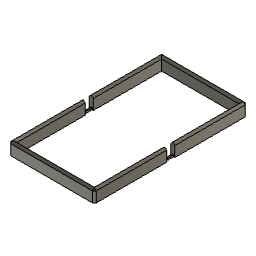
Sifting_Litter_Box_Spacer v3_30mm (Autodesk Fusion 360 design; units mm, degrees)
Autodesk Fusion 360 part; units mm, degrees
sketch "Sketch1" plane through (0, 0, 0) normal (0, 0, 1) x (1, 0, 0)
  line L0 (0, 0) -> (210, 0)
  line L1 (210, 0) -> (210, 355)
  line L2 (210, 355) -> (0, 355)
  line L3 (0, 355) -> (0, 0)
  line L4 (10, 345) -> (10, 10)
  line L5 (10, 10) -> (200, 10)
  line L6 (200, 10) -> (200, 345)
  line L7 (200, 345) -> (10, 345)
  dimension "d4" = 210
  dimension "d5" = 355
  constraint horizontal L0
  constraint vertical L1
  constraint horizontal L2
  constraint vertical L3
  constraint coincident L0.start L3.end
  measures "d4" distance of L0.start L0.end
  measures "d5" distance of L0.start L2.end
extrude "Extrude1" add sketch "Sketch1" along normal blind 30 makes body 1
chamfer "Chamfer1" distance 4.5 angle 45 4 edges at (10, 177.5, 30) (105, 10, 30) (200, 177.5, 30) (105, 345, 30) measured on face at (3.3333, 233.3333, 30) measured on face at (3.3333, 233.3333, 30) measured on face at (3.3333, 233.3333, 30) measured on face at (3.3333, 233.3333, 30) on bodies 1
ref_plane "WorkPlane1" through (105, 177.5, 15) normal (0, -1, 0) x (1, 0, 0)
split "Split1" by plane through (105, 177.5, 15) normal (0, -1, 0) bodies 1 makes body 2 at (70, 0, 10)
move_body "Move1" bodies 1 to x (1, 0, 0) y (0, 1, 0) z (0, 0, 1) at (0, 10, 0)
move_body "Move2" bodies 2 to x (1, 0, 0) y (0, 1, 0) z (0, 0, 1) at (0, -10, 0)
chamfer "Chamfer2" distance 4.5 angle 45 6 edges at (105, 365, 30) (0, 276.25, 30) (210, 276.25, 30) (0, 78.75, 30) (210, 78.75, 30) (105, -10, 30) 6 faces at (140, 365, 10) (0, 305.8333, 20) (210, 246.6667, 20) (0, 108.3333, 20) (210, 49.1667, 20) (70, -10, 10) measured on face at (71.8333, 363.1667, 30) measured on face at (71.8333, 363.1667, 30) measured on face at (71.8333, 363.1667, 30) measured on face at (71.8333, -8.1667, 30) measured on face at (71.8333, -8.1667, 30) measured on face at (71.8333, -8.1667, 30) on bodies 1 2
delete_face "DeleteFace1" 1 faces at (207, 166, 11.5) on bodies 2
delete_face "DeleteFace2" 1 faces at (207, 189, 18.5) on bodies 1
delete_face "DeleteFace3" 1 faces at (3, 189, 18.5) on bodies 1
delete_face "DeleteFace4" 1 faces at (3, 166, 11.5) on bodies 2
delete_face "DeleteFace5" 2 faces at (1.5, 245.1667, 3) (1.5, 52.1667, 3) on bodies 1 2
delete_face "DeleteFace6" 4 faces at (207, 362, 3) (208.5, 302.8333, 3) (207, 109.8333, 1.5) (207, -7, 3) on bodies 1 2
delete_face "DeleteFace7" 1 faces at (140, 362, 1.5) on bodies 1
delete_face "DeleteFace8" 1 faces at (140, -7, 1.5) on bodies 2
delete_face "DeleteFace9" 1 faces at (4.5, 362, 1.5) on bodies 1
delete_face "DeleteFace10" 1 faces at (3, -5.5, 1.5) on bodies 2
delete_face "DeleteFace11" 1 faces at (71.8333, 360.1667, 30) on bodies 1
delete_face "DeleteFace12" 1 faces at (138.1667, -5.1667, 30) on bodies 2
sketch "Sketch2" plane through (0, 187.5, 0) normal (0, -1, 0) x (1, 0, 0)
  line L0 (0, 0) -> (10, 0)
  line L1 (10, 0) -> (10, 25.5)
  line L2 (10, 25.5) -> (5, 30.5)
  line L3 (5, 30.5) -> (0, 25.5)
  line L4 (0, 25.5) -> (0, 0)
  line L5 (3, 0) -> (7, 0)
  line L6 (7, 0) -> (7, 4)
  line L7 (7, 4) -> (3, 4)
  line L8 (3, 4) -> (3, 0)
  dimension "d26" = 4
  dimension "d27" = 4
  constraint horizontal L5
  constraint vertical L6
  constraint horizontal L7
  constraint vertical L8
  constraint coincident L0 L5.start
  measures "d26" distance of L5.start L5.end
  measures "d27" distance of L5.start L7.end
extrude "Extrude2" cut sketch "Sketch2" against normal blind 20 contours L0 L5 L6 L7 L8 bodies 1
sketch "Sketch3" plane through (0, 167.5, 0) normal (0, 1, 0) x (-1, 0, 0)
  line L0 (0, 0) -> (0, 25.5)
  line L1 (0, 25.5) -> (-5, 30.5)
  line L2 (-5, 30.5) -> (-10, 25.5)
  line L3 (-10, 25.5) -> (-10, 0)
  line L4 (-10, 0) -> (0, 0)
  line L5 (-7, 0) -> (-3.2, 0)
  line L6 (-3.2, 0) -> (-3.2, 3.8)
  line L7 (-3.2, 3.8) -> (-7, 3.8)
  line L8 (-7, 3.8) -> (-7, 0)
  dimension "d30" = 3.8
  dimension "d31" = 3.8
  constraint horizontal L5
  constraint vertical L6
  constraint horizontal L7
  constraint vertical L8
  constraint coincident L4 L5.start
  measures "d30" distance of L5.start L5.end
  measures "d31" distance of L5.start L7.end
extrude "Extrude3" add sketch "Sketch3" along normal blind 20 contours L4 L5 L6 L7 L8 bodies 2
sketch "Sketch4" plane through (0, 187.5, 0) normal (0, -1, 0) x (1, 0, 0)
  line L0 (210, 0) -> (210, 25.5)
  line L1 (210, 25.5) -> (205, 30.5)
  line L2 (205, 30.5) -> (200, 25.5)
  line L3 (200, 25.5) -> (200, 0)
  line L4 (200, 0) -> (210, 0)
  line L5 (203, 0) -> (206.8, 0)
  line L6 (206.8, 0) -> (206.8, 3.8)
  line L7 (206.8, 3.8) -> (203, 3.8)
  line L8 (203, 3.8) -> (203, 0)
  dimension "d34" = 3.8
  dimension "d35" = 3.8
  constraint horizontal L5
  constraint vertical L6
  constraint horizontal L7
  constraint vertical L8
  constraint coincident L4 L5.start
  measures "d34" distance of L5.start L5.end
  measures "d35" distance of L5.start L7.end
extrude "Extrude4" add sketch "Sketch4" along normal blind 20 contours L4 L5 L6 L7 L8 bodies 1
sketch "Sketch5" plane through (0, 167.5, 0) normal (0, 1, 0) x (-1, 0, 0)
  line L0 (-210, 0) -> (-200, 0)
  line L1 (-200, 0) -> (-200, 25.5)
  line L2 (-200, 25.5) -> (-205, 30.5)
  line L3 (-205, 30.5) -> (-210, 25.5)
  line L4 (-210, 25.5) -> (-210, 0)
  line L5 (-207, 0) -> (-203, 0)
  line L6 (-203, 0) -> (-203, 4)
  line L7 (-203, 4) -> (-207, 4)
  line L8 (-207, 4) -> (-207, 0)
  dimension "d38" = 4
  dimension "d39" = 4
  constraint horizontal L5
  constraint vertical L6
  constraint horizontal L7
  constraint vertical L8
  constraint coincident L0 L5.start
  measures "d38" distance of L5.start L5.end
  measures "d39" distance of L5.start L7.end
extrude "Extrude5" cut sketch "Sketch5" against normal blind 20 contours L0 L5 L6 L7 L8 bodies 2
equation "Inner_Width = 210 mm"
equation "Inner_Length = 355 mm"
equation "Height = 30 mm"
equation "d4 = Inner_Width"
equation "d5 = Inner_Length"
equation "Thickness = 10 mm"
equation "d7 = -Thickness"
equation "d8 = Height"
equation "Inner_Chamfer = 4.5 mm"
equation "Inner_Chamfer_Angle = 45 deg"
equation "d12 = Inner_Chamfer"
equation "d13 = Inner_Chamfer_Angle"
equation "Outer_Chamfer = 4.5 mm"
equation "Outer_Chamfer_Angle = 45 deg"
equation "d17 = Outer_Chamfer"
equation "d18 = Outer_Chamfer_Angle"
equation "pin_depth = 20 mm"
equation "pin_diameter = 4 mm"
equation "pin_tolerance = 0.2 mm"
equation "d26 = pin_diameter"
equation "d27 = pin_diameter"
equation "d28 = -pin_depth"
equation "d30 = pin_diameter - pin_tolerance"
equation "d31 = pin_diameter - pin_tolerance"
equation "d32 = pin_depth"
equation "d34 = pin_diameter - pin_tolerance"
equation "d35 = pin_diameter - pin_tolerance"
equation "d36 = pin_depth"
equation "d38 = pin_diameter"
equation "d39 = pin_diameter"
equation "d40 = -pin_depth"
